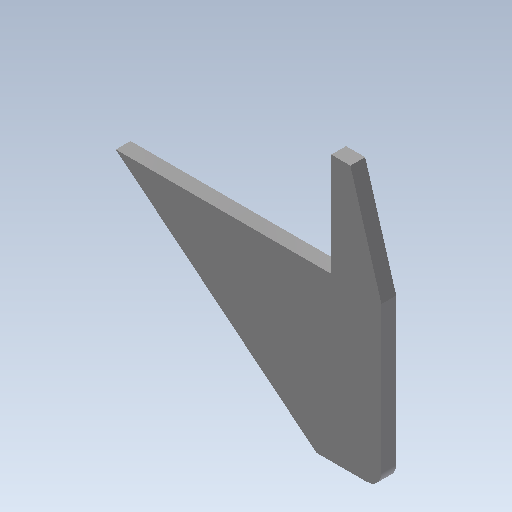
# Autodesk Inventor part: ADSK-MH-10039
Saved by Autodesk Inventor 2020.2 (Build 242310000, 310)
## iProperties
Created: 2008-03-27
Part Number: ADSK-MH-10039
Document SubType Name: Modeling
Designer: R.O'mahony
Density: 7.86 g/cm^3
Mass: 136.916 g
Surface Area: 85.3438 cm^2
Volume: 17.4193 cm^3
Material: Steel, Mild
Appearance: Steel
Description: Bracket Back Support-trans
Engineer: Demir Ali
Checked By: Demir Ali
Company: Autodesk Ltd
Author: R.O'mahony
Keywords: Roller Conveyor
Revision Number: A
Autodesk Inventor part; units mm, degrees
ref_plane "YZ Plane" through (0, 0, 0) normal (1, 0, 0) x (0, 1, 0)
ref_plane "XZ Plane" through (0, 0, 0) normal (0, 1, 0) x (-1, 0, 0)
ref_plane "XY Plane" through (0, 0, 0) normal (0, 0, 1) x (1, 0, 0)
sketch "Sketch1" plane through (0, 0, 0) normal (0, 0, 1) x (1, 0, 0)
  line L0 (2530.7582, -564.6941) -> (2513.7582, -564.6941)
  line L1 (2513.7582, -564.6941) -> (2445.7582, -509.6941)
  line L2 (2518.7582, -474.6941) -> (2518.7582, -509.6941)
  line L3 (2518.7582, -509.6941) -> (2445.7582, -509.6941)
  line L4 (2525.2455, -474.6941) -> (2535.7582, -510.0365)
  arc A0 (2530.7582, -564.6941) -> (2535.7582, -559.6941) centre (2530.7582, -559.6941) ccw
  line L5 (2525.2455, -474.6941) -> (2518.7582, -474.6941)
  line L6 (2535.7582, -559.6941) -> (2535.7582, -510.0365)
  arc A1 (2530.7582, -564.6941) -> (2535.7582, -559.6941) centre (2530.7582, -559.6941) ccw
  point P0 (0, 0)
  dimension "d2" = 90
  constraints: 14 end point, 4 point on circle, 2 centre point
  measures "d2" distance between parallel lines of L5 L0
extrude "Extrusion1" add sketch "Sketch1" along normal mid plane 5
body "Solid1"
